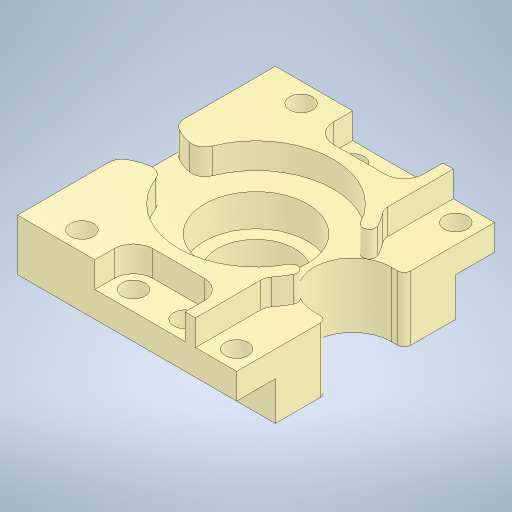
# Autodesk Inventor part: Spring Mount
Saved by Autodesk Inventor 2023.4 (Build 274418000, 418)
## iProperties
Created: 2024-03-24
Part Number: Spring Mount
Material: Nylon 6/6
Document SubType Name: Modeling
Designer: Nathan Cai
Density: 1.13 g/cm^3
Appearance: Nylon 6
Mass: 7.28213 g
Surface Area: 52.3259 cm^2
Volume: 6.44437 cm^3
Author: Nathan Cai
Autodesk Inventor part; units mm, degrees
ref_plane "YZ Plane" through (0, 0, 0) normal (1, 0, 0) x (0, 1, 0)
ref_plane "XZ Plane" through (0, 0, 0) normal (0, 1, 0) x (-1, 0, 0)
ref_plane "XY Plane" through (0, 0, 0) normal (0, 0, 1) x (1, 0, 0)
sketch "Sketch1" plane through (0, 0, 0) normal (0, 1, 0) x (-1, 0, 0)
  line L0 (-13.4938, 15.875) -> (13.4937, 15.875)
  line L1 (13.4937, 15.875) -> (13.4937, -15.875)
  line L2 (13.4937, -15.875) -> (-13.4938, -15.875)
  line L3 (-13.4938, -15.875) -> (-13.4938, 15.875)
  line L4 (-13.4938, 15.875) -> (13.4937, -15.875) construction
  line L5 (13.4937, 15.875) -> (-13.4938, -15.875) construction
  circle A0 centre (0, 0) radius 4.7625
  circle A1 centre (9.525, 8.7313) radius 6.35 construction
  line L6 (13.4937, 0) -> (-13.4938, 0) construction
  circle A2 centre (9.525, 8.7313) radius 1.7526
  circle A3 centre (9.525, -8.7312) radius 6.35 construction
  circle A4 centre (9.525, -8.7312) radius 1.7526
  dimension "d0" = 26.9875
  dimension "d1" = 31.75
  dimension "d2" = 9.525
  dimension "d3" = 12.7
  dimension "d4" = 3.5052
  dimension "d7" = 8.7312
  dimension "d8" = 3.9688
  constraints: 14 end point, 5 centre point, 4 midpoint, 2 coincident, 2 parallel, 2 symmetric about line, 1 horizontal, 1 perpendicular, 2 other
  measures "d0" distance of L1.end L2.end
  measures "d1" distance of L0.end L1.end
  measures "d2" diameter of A0
  measures "d3" diameter of A1
  measures "d4" diameter of A2
  measures "d7" distance from line of L6 A2.centre
  measures "d8" distance from line of L1 A2.centre
extrude "Extrusion1" add sketch "Sketch1" along normal blind 3.175
sketch "Sketch2" plane through (0, 3.175, 0) normal (0, 1, 0) x (1, 0, 0)
  circle A0 centre (0, 0) radius 9.525
  circle A1 centre (-9.525, 8.7312) radius 1.7526 projected
  circle A2 centre (-9.525, 8.7312) radius 6.35
  line L0 (13.4938, 15.875) -> (-13.4937, 15.875) projected
  line L1 (-13.4937, 15.875) -> (-13.4937, -15.875) projected
  line L2 (-13.4937, -15.875) -> (13.4938, -15.875) projected
  line L3 (13.4938, -15.875) -> (13.4938, 15.875) projected
  circle A3 centre (-9.525, 8.7312) radius 1.7526 projected
  circle A4 centre (-9.525, -8.7313) radius 1.7526 projected
  circle A5 centre (0, 0) radius 4.7625 projected
  circle A6 centre (-9.525, -8.7313) radius 6.35
  point P0 (-13.4937, 13.6882)
  point P1 (-13.4937, 3.7743)
  point P2 (-9.2207, 2.3885)
  point P3 (-3.1798, 8.9786)
  point P4 (-9.2207, -2.3885)
  point P5 (-13.4937, -3.7743)
  point P6 (-13.4937, -13.6882)
  point P7 (-3.1798, -8.9786)
  dimension "d9" = 19.05
  dimension "d10" = 12.7
  dimension "d11" = 12.7
  constraints: 3 centre point, 3 coincident
  measures "d9" diameter of A0
  measures "d10" diameter of A2
  measures "d11" diameter of A6
extrude "Extrusion2" add sketch "Sketch2" along normal blind 3.175 contours A0 A2 L1 L0 L3 L2 A6 | A0 A2 L1 | A6 L1 A0 | A1 | A4
sketch "Sketch4" plane through (0, 0, 0) normal (0, -1, 0) x (1, 0, 0)
  line L0 (-13.4937, -3.7743) -> (-13.4937, 3.7743) projected
  line L1 (-13.4937, 13.4938) -> (13.4938, 13.4937) construction
  line L2 (13.4938, 15.875) -> (13.4938, -15.875) projected
  line L3 (-13.4937, 15.875) -> (13.4938, 15.875) projected
  circle A0 centre (-7.9375, 13.4938) radius 1.4224
  circle A1 centre (-1.5875, 13.4937) radius 1.4224
  circle A2 centre (4.7625, 13.4937) radius 1.4224
  circle A3 centre (11.1125, 13.4937) radius 1.4224
  line L4 (-13.4937, -3.7743) -> (-13.4937, 3.7743) projected
  line L5 (-13.4937, 0) -> (13.4938, 0) construction
  line L6 (-13.4938, -13.4937) -> (13.4938, -13.4937) construction
  circle A4 centre (-7.9375, -13.4938) radius 1.4224
  circle A5 centre (-1.5875, -13.4938) radius 1.4224
  circle A6 centre (4.7625, -13.4937) radius 1.4224
  circle A7 centre (11.1125, -13.4937) radius 1.4224
  point P0 (0, 0)
  point P1 (-13.4937, 12.8557)
  point P2 (-13.4937, -4.6068)
  point P3 (-13.4937, 4.6068)
  dimension "d19" = 2.3813
  dimension "d20" = 2.8448
  dimension "d21" = 5.5563
  dimension "d24" = 6.35
  constraints: 8 centre point, 6 end point, 6 symmetric about line, 4 point on line, 2 midpoint, 1 horizontal, 1 parallel, 10 other
  measures "d19" distance between parallel lines of L3 L1
  measures "d20" diameter of A0
  measures "d21" distance from line of L0 A0.centre
  measures "d24" distance of A0.centre A1.centre
extrude "Extrusion4" cut sketch "Sketch4" against normal through all
sketch "Sketch5" plane through (0, 6.35, 0) normal (0, 1, 0) x (1, 0, 0)
  line L0 (13.4938, -15.875) -> (13.4938, 15.875) projected
  line L1 (13.4938, 0) -> (-13.4937, 0) construction
  line L2 (-13.4937, 15.875) -> (-13.4937, -15.875) projected
  line L3 (4.7625, -13.4937) -> (-1.5875, -13.4937) construction
  line L4 (4.7625, -11.1125) -> (-1.5875, -11.1125)
  line L5 (-1.5875, -15.875) -> (4.7625, -15.875)
  arc A0 (4.7625, -15.875) -> (4.7625, -11.1125) centre (4.7625, -13.4937) ccw
  arc A1 (-1.5875, -11.1125) -> (-1.5875, -15.875) centre (-1.5875, -13.4937) ccw
  line L6 (-13.4937, -15.875) -> (13.4938, -15.875) projected
  line L7 (7.1438, -13.4937) -> (-3.9687, -13.4937) construction
  line L8 (-3.9687, -13.4937) -> (-3.9687, -15.875)
  line L9 (-3.9687, -15.875) -> (7.1438, -15.875)
  line L10 (7.1438, -15.875) -> (7.1438, -13.4937)
  line L11 (4.7625, 13.4937) -> (-1.5875, 13.4937) construction
  line L12 (4.7625, 11.1125) -> (-1.5875, 11.1125)
  line L13 (-1.5875, 15.875) -> (4.7625, 15.875)
  arc A2 (4.7625, 11.1125) -> (4.7625, 15.875) centre (4.7625, 13.4937) ccw
  arc A3 (-1.5875, 15.875) -> (-1.5875, 11.1125) centre (-1.5875, 13.4937) ccw
  line L14 (7.1437, 13.4937) -> (-3.9688, 13.4937) construction
  line L15 (-3.9688, 13.4937) -> (-3.9688, 15.875)
  line L16 (-3.9688, 15.875) -> (7.1437, 15.875)
  line L17 (7.1437, 15.875) -> (7.1437, 13.4937)
  circle A4 centre (4.7625, -13.4937) radius 1.4224 projected
  circle A5 centre (-1.5875, -13.4937) radius 1.4224 projected
  point P0 (0, 0)
  point P1 (1.5875, -13.4937)
  point P2 (1.5875, 13.4937)
  point P3 (-3.9687, 13.4937)
  point P4 (-3.9687, -13.4937)
  point P5 (7.1438, -15.875)
  constraints: 34 end point, 11 symmetric about line, 9 point on circle, 5 tangent, 4 centre point, 3 midpoint, 3 parallel, 2 concentric, 2 horizontal, 2 point on line, 1 perpendicular, 2 other
extrude "Extrusion5" cut sketch "Sketch5" along normal blind 25.4 and the other way blind 3.175 contours A0 L5 A1 L4 | L10 L6 A0 | A1 L6 L8 | L12 A3 L13 A2 | A2 L16 L17 | L15 L16 A3 | A4 | A5
fillet "Fillet3" radius 1.5875 4 edges at (-9.2207, 4.7625, 2.3885) (-9.2207, 4.7625, -2.3885) (-13.4937, 4.7625, -3.7743) (-13.4937, 4.7625, 3.7743)
sketch "Sketch6" plane through (0, 6.35, 0) normal (0, 1, 0) x (1, 0, 0)
  line L0 (13.4938, -15.875) -> (13.4938, 15.875) projected
  circle A0 centre (0, 0) radius 11.1125
  line L1 (7.1438, -15.875) -> (13.4938, -15.875) projected
  line L2 (8.422, -15.875) -> (8.422, -7.2497)
  line L3 (0, 0) -> (11.1125, 0) construction
  line L4 (7.1438, -13.4937) -> (7.1438, -15.875) projected
  line L5 (8.422, 15.875) -> (8.422, 7.2497)
  line L6 (7.1437, 15.875) -> (7.1437, 13.4937) projected
  arc A1 (4.7625, 11.1125) -> (7.1437, 13.4937) centre (4.7625, 13.4937) ccw projected
  line L7 (4.7625, 11.1125) -> (-1.5875, 11.1125) projected
  arc A2 (-3.9687, 13.4937) -> (-1.5875, 11.1125) centre (-1.5875, 13.4937) ccw projected
  arc A3 (-8.8729, -3.4638) -> (-8.8729, 3.4638) centre (0, 0) ccw projected
  arc A4 (-1.5875, -11.1125) -> (-3.9687, -13.4937) centre (-1.5875, -13.4937) ccw projected
  line L8 (-1.5875, -11.1125) -> (4.7625, -11.1125) projected
  arc A5 (7.1438, -13.4937) -> (4.7625, -11.1125) centre (4.7625, -13.4937) ccw projected
  line L9 (7.1438, -13.4937) -> (7.1438, -15.875) projected
  line L10 (7.1438, -15.875) -> (13.4938, -15.875) projected
  line L11 (13.4938, -15.875) -> (13.4938, 15.875) projected
  line L12 (13.4938, 15.875) -> (7.1437, 15.875) projected
  line L13 (-3.9687, 13.4937) -> (-3.9688, 15.875) projected
  line L14 (-3.9688, 15.875) -> (-13.4937, 15.875) projected
  line L15 (-13.4937, 15.875) -> (-13.4937, 4.6068) projected
  circle A6 centre (-7.9375, 13.4938) radius 1.4224 projected
  arc A7 (-10.6273, 2.4776) -> (-8.8729, 3.4638) centre (-10.3517, 4.041) ccw projected
  line L16 (-13.4937, -4.6068) -> (-13.4937, -15.875) projected
  arc A8 (-13.4937, 4.6068) -> (-12.7, 3.232) centre (-11.9062, 4.6068) ccw projected
  arc A9 (-12.7, 3.232) -> (-10.6273, 2.4776) centre (-9.525, 8.7312) ccw projected
  circle A10 centre (-7.9375, -13.4938) radius 1.4224 projected
  line L17 (-13.4937, -15.875) -> (-3.9687, -15.875) projected
  line L18 (-3.9687, -15.875) -> (-3.9687, -13.4937) projected
  arc A11 (-8.8729, -3.4638) -> (-10.6273, -2.4776) centre (-10.3517, -4.041) ccw projected
  arc A12 (-10.6273, -2.4776) -> (-12.7, -3.232) centre (-9.525, -8.7313) ccw projected
  arc A13 (-12.7, -3.232) -> (-13.4937, -4.6068) centre (-11.9062, -4.6068) ccw projected
  point P0 (8.422, 15.875)
  point P1 (8.422, 7.2497)
  point P2 (3.9688, -14.6741)
  dimension "d42" = 22.225
  dimension "d43" = 1.2782
  constraints: 6 end point, 2 perpendicular, 2 point on circle, 2 symmetric about line, 1 centre point, 1 coincident, 1 point on line, 1 other
  measures "d42" diameter of A0
extrude "Extrusion6" cut sketch "Sketch6" against normal blind 3.175 contours L1 L2 A0 L5 L12 L0
fillet "Fillet4" radius 1.5875 2 edges at (8.422, 4.7625, -7.2497) (8.422, 4.7625, 7.2497)
sketch "Sketch7" plane through (0, 0, 0) normal (0, -1, 0) x (1, 0, 0)
  line L0 (13.4938, 15.875) -> (13.4938, -15.875) projected
  line L1 (-13.4938, -11.1125) -> (13.4938, -11.1125)
  line L2 (13.4938, -11.1125) -> (13.4938, 11.1125)
  line L3 (13.4938, 11.1125) -> (-13.4938, 11.1125)
  line L4 (-13.4938, 11.1125) -> (-13.4938, -11.1125)
  line L5 (-13.4938, -11.1125) -> (13.4938, 11.1125) construction
  line L6 (13.4938, -11.1125) -> (-13.4938, 11.1125) construction
  line L7 (-13.4937, 15.875) -> (13.4938, 15.875) projected
  line L8 (0, 0) -> (0, 9.525) construction
  circle A0 centre (-1.5875, 13.4937) radius 1.4224 projected
  circle A1 centre (-1.5875, -13.4938) radius 1.4224 projected
  circle A2 centre (-7.9375, -13.4938) radius 1.4224 projected
  circle A3 centre (-7.9375, 13.4938) radius 1.4224 projected
  circle A4 centre (4.7625, 13.4937) radius 1.4224 projected
  circle A5 centre (4.7625, -13.4937) radius 1.4224 projected
  line L9 (13.4938, -15.875) -> (-13.4937, -15.875) projected
  line L10 (-13.4937, 15.875) -> (13.4938, 15.875) projected
  line L11 (-13.4937, -15.875) -> (-13.4937, 15.875) projected
  circle A6 centre (-9.525, -8.7312) radius 1.7526 projected
  circle A7 centre (-9.525, 8.7313) radius 1.7526 projected
  circle A8 centre (0, 0) radius 4.7625 projected
  line L12 (13.4938, 15.875) -> (13.4938, -15.875) projected
  dimension "d45" = 4.7625
  constraints: 14 end point, 2 midpoint, 2 parallel, 1 horizontal, 1 perpendicular, 1 point on line, 1 vertical
  measures "d45" distance between parallel lines of L7 L3
extrude "Extrusion7" add sketch "Sketch7" along normal blind 4.7625 contours L0 L1 L4 L3 | A6 | A7
sketch "Sketch8" plane through (0, -4.7625, 0) normal (0, -1, 0) x (1, 0, 0)
  line L0 (15.0813, 0) -> (11.9063, 0) construction
  line L1 (13.4938, -11.1125) -> (13.4938, 11.1125) projected
  line L2 (15.0813, 4.7625) -> (11.9063, 4.7625)
  line L3 (11.9063, -4.7625) -> (15.0813, -4.7625)
  arc A0 (15.0813, -4.7625) -> (15.0813, 4.7625) centre (15.0813, 0) ccw
  arc A1 (11.9063, 4.7625) -> (11.9063, -4.7625) centre (11.9063, 0) ccw
  point P0 (0, 0)
  point P1 (13.4938, 0)
  point P2 (13.4938, -4.7625)
  point P3 (13.4938, 4.7625)
  dimension "d57" = 9.525
  dimension "d58" = 3.175
  constraints: 8 end point, 4 point on circle, 4 tangent, 2 centre point, 2 midpoint, 1 horizontal, 1 parallel
  measures "d57" diameter of A1
  measures "d58" distance of L0.end L0.start
extrude "Extrusion8" cut sketch "Sketch8" against normal through all contours L3 A1 L2 L1
fillet "Fillet6" radius 0.7937 6 edges at (8.8106, 4.7625, -3.6192) (10.1865, 4.7625, -4.4411) (10.1865, 4.7625, 4.4411) (8.8106, 4.7625, 3.6192) (13.4938, -0.7938, 4.7625) (13.4938, -0.7938, -4.7625)
sketch "Sketch10" plane through (0, -4.7625, 0) normal (0, -1, 0) x (1, 0, 0)
  circle A0 centre (0, 0) radius 8 construction
  circle A1 centre (0, 0) radius 9.5 construction
  line L0 (0, 0) -> (-6.7175, -6.7175) construction
  line L1 (0, 0) -> (-6.7175, 6.7175) construction
  line L2 (0, 8) -> (0, 0) construction
  circle A2 centre (-6.7175, -6.7175) radius 2.75
  circle A3 centre (-5.6569, 5.6569) radius 2.75
  circle A4 centre (6.7175, 6.7175) radius 2.75
  circle A5 centre (5.6569, -5.6569) radius 2.75
  dimension "d71" = 16
  dimension "d72" = 19
  dimension "d73" = 45
  dimension "d74" = 5.5
  dimension "d75" = 5.5
  dimension "d78" = 360
  constraints: 6 centre point, 6 end point, 5 point on circle, 2 coincident, 2 point on line, 1 perpendicular, 1 vertical, 9 other
  measures "d71" diameter of A0
  measures "d72" diameter of A1
  measures "d73" angle of L2 L1
  measures "d74" diameter of A2
  measures "d75" diameter of A3
extrude "Extrusion10" cut sketch "Sketch10" against normal blind 4
chamfer "Chamfer1" distance 1 angle 45 4 edges at (-9.4675, -0.7625, -6.7175) (-8.4069, -0.7625, 5.6569) (2.9069, -0.7625, -5.6569) (3.9675, -0.7625, 6.7175)
sketch "Sketch11" plane through (0, 3.175, 0) normal (0, 1, 0) x (1, 0, 0)
  circle A0 centre (0, 0) radius 6.35
  dimension "d85" = 12.7
  constraints: 1 centre point, 1 coincident
  measures "d85" diameter of A0
extrude "Extrusion11" cut sketch "Sketch11" against normal blind 3.9688
equation "\"d11\" = d10"
body "Solid1"
